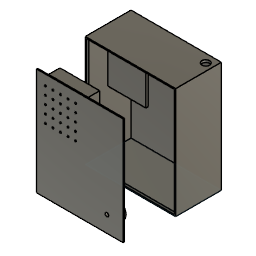
WalkieTalkie (Autodesk Fusion 360 design; units mm, degrees)
part number: 2026-07-24-17-12-39-216
Autodesk Fusion 360 part; units mm, degrees
sketch "Szkic1" plane through (0, 0, 0) normal (0, 1, 0) x (1, 0, 0)
  line L0 (0, 0) -> (75, 0)
  line L1 (75, 0) -> (75, -92)
  line L2 (75, -92) -> (0, -92)
  line L3 (0, -92) -> (0, 0)
  dimension "d1" = 75
  dimension "d2" = 92
  constraint horizontal L0
  constraint vertical L1
  constraint horizontal L2
  constraint vertical L3
  constraint coincident L0.start L3.end
  measures "d1" distance of L0.start L0.end
  measures "d2" distance of L0.start L2.end
extrude "Wyciągnięcie proste1" add sketch "Szkic1" along normal blind 38 makes body 1
shell "Skorupa1" thickness 2 removed faces 1 at (25, 0, 61.3333) on bodies 1
sketch "Szkic6" plane through (0, 0, 0) normal (0, -1, 0) x (1, 0, 0)
  line L0 (2, 2) -> (2, 90)
  line L1 (2, 90) -> (73, 90)
  line L2 (73, 90) -> (73, 2)
  line L3 (73, 2) -> (2, 2)
  line L4 (75, 92) -> (0, 92)
  line L5 (0, 92) -> (0, 0)
  line L6 (0, 0) -> (75, 0)
  line L7 (75, 0) -> (75, 92)
  line L8 (73.5, 90.5) -> (1.5, 90.5)
  line L9 (1.5, 90.5) -> (1.5, 1.5)
  line L10 (1.5, 1.5) -> (73.5, 1.5)
  line L11 (73.5, 1.5) -> (73.5, 90.5)
  dimension "d8" = -1.5
extrude "Wyciągnięcie proste2" add sketch "Szkic6" along normal blind 2 separate body contours L0 L1 L2 L3 | L8 L9 L10 L11 makes body 2
sketch "Szkic7" plane through (0, 0, 0) normal (0, 1, 0) x (-1, 0, 0)
  line L0 (-73.5, 90.5) -> (-73.5, 1.5)
  line L1 (-73.5, 1.5) -> (-1.5, 1.5)
  line L2 (-1.5, 1.5) -> (-1.5, 90.5)
  line L3 (-1.5, 90.5) -> (-73.5, 90.5)
  line L4 (-5, 85) -> (-38, 85)
  line L5 (-38, 85) -> (-38, 52)
  line L6 (-38, 52) -> (-5, 52)
  line L7 (-5, 52) -> (-5, 85)
  line L8 (-37.25, 52.75) -> (-5.75, 52.75)
  line L9 (-5.75, 52.75) -> (-5.75, 84.25)
  line L10 (-5.75, 84.25) -> (-37.25, 84.25)
  line L11 (-37.25, 84.25) -> (-37.25, 52.75)
  dimension "d11" = 33
  dimension "d12" = 33
  dimension "d13" = -0.75
  constraint horizontal L4
  constraint vertical L5
  constraint horizontal L6
  constraint vertical L7
  measures "d11" distance of L4.start L4.end
  measures "d12" distance of L4.start L6.end
extrude "Wyciągnięcie proste3" add sketch "Szkic7" along normal blind 14 contours L4 L5 L6 L7 bodies 2
sketch "Szkic8" plane through (0, 14, 0) normal (0, 1, 0) x (-1, 0, 0)
  line L0 (-37.25, 52.75) -> (-37.25, 84.25)
  line L1 (-37.25, 84.25) -> (-5.75, 84.25)
  line L2 (-5.75, 84.25) -> (-5.75, 52.75)
  line L3 (-5.75, 52.75) -> (-37.25, 52.75)
  line L4 (-5, 52) -> (-5, 85)
  line L5 (-5, 85) -> (-38, 85)
  line L6 (-38, 85) -> (-38, 52)
  line L7 (-38, 52) -> (-5, 52)
  line L8 (-37.25, 52.75) -> (-5, 52.75)
  line L9 (-5, 52.75) -> (-5, 85)
  line L10 (-5, 85) -> (-37.25, 85)
  line L11 (-37.25, 85) -> (-37.25, 52.75)
  constraint horizontal L8
  constraint vertical L9
  constraint horizontal L10
  constraint vertical L11
  constraint coincident L4.end L5.start
  constraint coincident L0.start L3.end
extrude "Wyciągnięcie proste4" add sketch "Szkic8" along normal blind 1 separate body contours L0 L1 L2 L3 L8 L11 makes body 3
move_body "Przesuń1" bodies 2 to x (1, 0, 0) y (0, 1, 0) z (0, 0, 1) at (0, -40, 0)
sketch "Szkic9" plane through (0, -42, 0) normal (0, -1, 0) x (1, 0, 0)
  line L0 (73.5, 1.5) -> (73.5, 90.5)
  line L1 (73.5, 90.5) -> (1.5, 90.5)
  line L2 (1.5, 90.5) -> (1.5, 1.5)
  line L3 (1.5, 1.5) -> (73.5, 1.5)
  circle A0 centre (9, 82) radius 0.75
  dimension "d18" = 1.5
  measures "d18" diameter of A0
extrude "Wyciągnięcie proste5" cut sketch "Szkic9" against normal blind 2 contours A0 bodies 2
pattern_linear "Szyk prostokątny1" count 5 spacing 6.25 along (1, 0, 0) count 5 spacing 6.75 along (0, 0, -1) of "Wyciągnięcie proste5"
sketch "Szkic10" plane through (0, -40, 0) normal (0, 1, 0) x (-1, 0, 0)
  line L0 (-73.5, 90.5) -> (-73.5, 1.5)
  line L1 (-73.5, 1.5) -> (-1.5, 1.5)
  line L2 (-1.5, 1.5) -> (-1.5, 90.5)
  line L3 (-1.5, 90.5) -> (-73.5, 90.5)
  line L4 (-5, 52) -> (-38, 52)
  line L5 (-38, 52) -> (-38, 85)
  line L6 (-38, 85) -> (-5, 85)
  line L7 (-5, 85) -> (-5, 52)
  circle A0 centre (-60, 15) radius 8
  dimension "d25" = 16
  measures "d25" diameter of A0
extrude "Wyciągnięcie proste6" add sketch "Szkic10" along normal blind 6 contours A0 bodies 2
sketch "Szkic11" plane through (0, -34, 0) normal (0, 1, 0) x (-1, 0, 0)
  circle A0 centre (-60, 15) radius 8
  circle A1 centre (-60, 15) radius 7.25
  dimension "d28" = 14.5
  constraint concentric A0 A1
  measures "d28" diameter of A1
extrude "Wyciągnięcie proste7" cut sketch "Szkic11" against normal blind 6 contours A1 bodies 2
sketch "Szkic12" plane through (0, -40, 0) normal (0, 1, 0) x (-1, 0, 0)
  circle A0 centre (-60, 15) radius 7.25
  circle A1 centre (-60, 15) radius 1.5
  dimension "d31" = 3
  constraint concentric A0 A1
  measures "d31" diameter of A1
extrude "Wyciągnięcie proste8" cut sketch "Szkic12" against normal blind 2 contours A1 bodies 2
sketch "Szkic13" plane through (0, 0, 0) normal (0, 0, -1) x (1, 0, 0)
  line L0 (75, 0) -> (0, 0)
  line L1 (0, 0) -> (0, -38)
  line L2 (0, -38) -> (75, -38)
  line L3 (75, -38) -> (75, 0)
sketch "Szkic14" plane through (0, 0, 0) normal (0, 0, -1) x (1, 0, 0)
sketch "Szkic15" plane through (0, 0, 0) normal (0, 0, -1) x (1, 0, 0)
  line L0 (65, -26.5) -> (56, -26.5)
  line L1 (56, -26.5) -> (56, -23)
  line L2 (56, -23) -> (65, -23)
  line L3 (65, -23) -> (65, -26.5)
  dimension "d36" = 9
  dimension "d37" = 3.5
  constraint horizontal L0
  constraint vertical L1
  constraint horizontal L2
  constraint vertical L3
  measures "d36" distance of L0.start L0.end
  measures "d37" distance of L0.start L2.end
extrude "Wyciągnięcie proste9" cut sketch "Szkic15" against normal blind 2 bodies 1
sketch "Szkic16" plane through (0, 0, 92) normal (0, 0, 1) x (-1, 0, 0)
  line L0 (0, 0) -> (-75, 0)
  line L1 (-75, 0) -> (-75, -38)
  line L2 (-75, -38) -> (0, -38)
  line L3 (0, -38) -> (0, 0)
  circle A0 centre (-69, -31) radius 3.25
  dimension "d40" = 6.5
  measures "d40" diameter of A0
extrude "Wyciągnięcie proste10" cut sketch "Szkic16" against normal blind 2 contours A0 bodies 1
sketch "Szkic17" plane through (0, 0, 0) normal (-1, 0, 0) x (0, -1, 0)
  line L0 (0, 0) -> (0, 92)
  line L1 (0, 92) -> (-38, 92)
  line L2 (-38, 92) -> (-38, 0)
  line L3 (-38, 0) -> (0, 0)
  circle A0 centre (-10, 33) radius 4.75
  dimension "d43" = 9.5
  measures "d43" diameter of A0
extrude "Wyciągnięcie proste11" cut sketch "Szkic17" against normal blind 2 contours A0 bodies 1
extrude "Wyciągnięcie proste12" add 1 faces at (16.25, 14, 63.25) along direction (0, -1, 0) blind 1 on bodies 3 bodies 3
chamfer "Fazowanie1" distance 1 angle 45 4 edges at (37.5, -40, 1.5) (73.5, -40, 46) (1.5, -40, 46) (37.5, -40, 90.5) on bodies 2
chamfer "Fazowanie2" distance 1 angle 45 4 edges at (37.5, 0, 2) (2, 0, 46) (37.5, 0, 90) (73, 0, 46) on bodies 1
moveface "Przesuń powierzchnię1" [suppressed]
